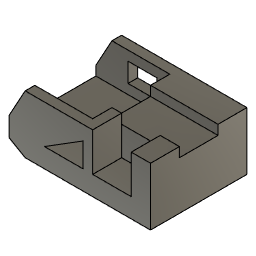
Sketch13_Final v0 (Autodesk Fusion 360 design; units mm, degrees)
Autodesk Fusion 360 part; units mm, degrees
sketch "Sketch1" plane through (0, 0, 0) normal (0, 1, 0) x (1, 0, 0)
  line L0 (0, 0) -> (39, 0)
  line L1 (0, 0) -> (-39, 0)
  line L2 (39, 0) -> (39, -36)
  line L3 (-39, -36) -> (39, -36)
  line L4 (-39, 0) -> (-49, -5.7735)
  line L5 (-39, 0) -> (1.8239, 0) construction
  line L6 (-49, -5.7735) -> (-49, -17.7735)
  line L7 (-49, -17.7735) -> (-39, -36)
  dimension "d1" = 39
  dimension "d2" = 39
  dimension "d4" = 36
  dimension "d5" = 36
  dimension "d8" = 12
  constraint coincident L0.start L1.start
  constraint horizontal L0
  constraint parallel L0 L1
  constraint perpendicular L0 L2
  constraint horizontal L5
  constraint vertical L6
  measures "d1" distance of L0.start L0.end
  measures "d2" distance of L0.start L1.end
  measures "d4" distance of L0.end L2.end
  measures "d5" distance of L1.end L3.start
  measures "d8" distance of L4.end L6.end
extrude "Extrude1" add sketch "Sketch1" along normal mid plane 60
sketch "Sketch2" plane through (0, 0, 0) normal (0, 0, 1) x (1, 0, 0)
  line L0 (39, -30) -> (39, -12)
  line L1 (39, -12) -> (39, 12)
  line L2 (33, -30) -> (9, -30)
  line L3 (33, -12) -> (9, -12)
  line L4 (9, -12) -> (9, -30)
  line L5 (39, 12) -> (-3, 12)
  line L6 (39, -12) -> (-3, -12)
  line L7 (-3, -12) -> (-3, 12)
  dimension "d11" = 18
  dimension "d12" = 24
  dimension "d13" = 24
  dimension "d14" = 42
  dimension "d15" = 42
  constraint vertical L0
  constraint vertical L1
  constraint perpendicular L0 L2
  constraint horizontal L3
  constraint perpendicular L1 L5
  constraint perpendicular L0 L6
  measures "d11" distance of L0.start L0.end
  measures "d12" distance of L0.end L1.end
  measures "d13" distance of L2.start L2.end
  measures "d14" distance of L1.end L5.end
  measures "d15" distance of L0.end L6.end
extrude "Extrude2" cut sketch "Sketch2" along normal blind 10 from surface at 30
sketch "Sketch3" plane through (0, 0, 0) normal (0, 0, 1) x (1, 0, 0)
  line L0 (27, -30) -> (3, -30)
  line L1 (27, -30) -> (27, -12)
  line L2 (3, -30) -> (3, -12)
  line L3 (3, -12) -> (27, -12)
  dimension "d20" = 24
  dimension "d21" = 18
  dimension "d22" = 18
  constraint horizontal L0
  constraint perpendicular L0 L2
  measures "d20" distance of L0.start L0.end
  measures "d21" distance of L0.start L1.end
  measures "d22" distance of L0.end L2.end
extrude "Extrude3" cut sketch "Sketch3" along normal blind 30 from surface at 12
sketch "Sketch4" plane through (0, 0, 0) normal (0, 0, 1) x (1, 0, 0)
  line L0 (-3, 12) -> (-3, 24)
  line L1 (-3, 30) -> (-40, 30)
  line L2 (-40, 24) -> (-3, 24)
  line L3 (-40, 24) -> (-49.0656, 24)
  line L4 (-3, -24) -> (-49, -24)
  line L5 (-3, -24) -> (-3, -12)
  line L6 (-3, -12) -> (-3, 12)
  line L7 (-49.0656, 24) -> (-49, -24)
  dimension "d27" = 6
  constraint perpendicular L0 L2
  constraint perpendicular L4 L5
  measures "d27" distance of L1.end L2.start
extrude "Extrude4" cut sketch "Sketch4" along normal blind 30 from surface at 12
sketch "Sketch5" plane through (0, 0, 0) normal (0, 1, 0) x (1, 0, 0)
  line L0 (-27, -12) -> (-3, -12)
  line L1 (-3, -12) -> (-3, -27)
  line L2 (-27, -12) -> (-3, -27)
  dimension "d34" = 24
  dimension "d35" = 15
  constraint perpendicular L0 L1
  measures "d34" distance of L0.start L0.end
  measures "d35" distance of L0.end L1.end
extrude "Extrude5" cut sketch "Sketch5" against normal blind 35
sketch "Sketch6" plane through (0, 0, 0) normal (0, 1, 0) x (1, 0, 0)
  line L0 (-29, -30) -> (-11, -30)
  line L1 (-29, -30) -> (-29, -18)
  line L2 (-11, -30) -> (-11, -18)
  line L3 (-11, -18) -> (-29, -18)
  dimension "d41" = 18
  dimension "d42" = 12
  dimension "d43" = 12
  constraint perpendicular L0 L1
  constraint perpendicular L0 L2
  constraint perpendicular L2 L3
  measures "d41" distance of L0.start L0.end
  measures "d42" distance of L0.start L1.end
  measures "d43" distance of L0.end L2.end
extrude "Extrude6" cut sketch "Sketch6" along normal blind 35
